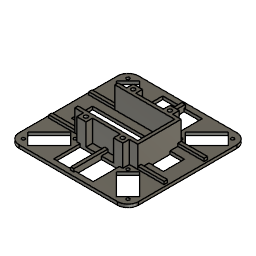
Spider_plate (Autodesk Fusion 360 design; units mm, degrees)
Autodesk Fusion 360 part; units mm, degrees
other "기준 메쉬 피쳐1"
sketch "스케치1" plane through (0, 0, 0) normal (0, 0, 1) x (1, 0, 0)
  line L0 (45.5, -45.5) -> (-45.5, -45.5)
  line L1 (-45.5, -45.5) -> (-45.5, 45.5)
  line L2 (-45.5, 45.5) -> (45.5, 45.5)
  line L3 (45.5, 45.5) -> (45.5, -45.5)
  line L4 (45.5, -45.5) -> (-45.5, 45.5) construction
  line L5 (-45.5, -45.5) -> (45.5, 45.5) construction
  line L6 (15, 41.5) -> (15, 21.5)
  line L7 (-15, 21.5) -> (-15, 41.5)
  line L8 (-1.25, 42.5) -> (1.25, 42.5)
  line L9 (1.25, 42.5) -> (1.25, 16.5)
  line L10 (1.25, 16.5) -> (-1.25, 16.5)
  line L11 (-1.25, 16.5) -> (-1.25, 42.5)
  line L12 (35, -8) -> (-35, -8)
  line L13 (-35, -8) -> (-35, 8)
  line L14 (-35, 8) -> (35, 8)
  line L15 (35, 8) -> (35, -8)
  line L16 (35, -8) -> (-35, 8) construction
  line L17 (-35, -8) -> (35, 8) construction
  line L18 (-15, 41.5) -> (-1.25, 41.5)
  line L19 (1.25, 41.5) -> (15, 41.5)
  line L20 (15, 21.5) -> (1.25, 21.5)
  line L21 (-1.25, 21.5) -> (-15, 21.5)
  line L22 (-44, 16.5) -> (44, 16.5)
  line L23 (44, 16.5) -> (44, 14)
  line L24 (-44, 14) -> (-44, 16.5)
  line L25 (-44, 16.5) -> (44, 16.5)
  line L26 (44, 16.5) -> (44, 14)
  line L27 (-44, 14) -> (-44, 16.5)
  line L28 (-17.4302, 26.1983) -> (-26.1983, 17.4302)
  line L29 (-26.1983, 17.4302) -> (-42.5325, 33.7643)
  line L30 (-42.5325, 33.7643) -> (-33.7643, 42.5325)
  line L31 (-33.7643, 42.5325) -> (-17.4302, 26.1983)
  line L32 (-17.4302, 26.1983) -> (-42.5325, 33.7643) construction
  line L33 (-26.1983, 17.4302) -> (-33.7643, 42.5325) construction
  circle A0 centre (-20.1172, 20.1172) radius 1.2
  circle A1 centre (-39.8455, 39.8455) radius 1.2
  line L34 (42.5325, 33.7643) -> (26.1983, 17.4302)
  line L35 (26.1983, 17.4302) -> (17.4302, 26.1983)
  line L36 (17.4302, 26.1983) -> (33.7643, 42.5325)
  line L37 (33.7643, 42.5325) -> (42.5325, 33.7643)
  circle A2 centre (39.8455, 39.8455) radius 1.2
  circle A3 centre (20.1172, 20.1172) radius 1.2
  line L38 (-24, 16.5) -> (-24, 14)
  line L39 (24, 16.5) -> (24, 14)
  line L40 (-17.5, 16.5) -> (-17.5, 21.5)
  line L41 (-15, 21.5) -> (-17.5, 21.5)
  line L42 (-10.5, 21.5) -> (-10.5, 16.5)
  circle A4 centre (-14, 18) radius 1.5
  line L43 (0, 42.5) -> (0, 16.5)
  line L44 (17.5, 16.5) -> (17.5, 21.5)
  line L45 (10.5, 21.5) -> (10.5, 16.5)
  line L46 (15, 21.5) -> (17.5, 21.5)
  circle A5 centre (14, 18) radius 1.5
  line L47 (-45.5, 0) -> (45.5, 0)
  circle A6 centre (14, -18) radius 1.5
  line L48 (1.25, -42.5) -> (1.25, -16.5)
  line L49 (-17.5, -16.5) -> (-17.5, -21.5)
  line L50 (-17.4302, -26.1983) -> (-42.5325, -33.7643) construction
  line L51 (-10.5, -21.5) -> (-10.5, -16.5)
  line L52 (15, -21.5) -> (17.5, -21.5)
  line L53 (-26.1983, -17.4302) -> (-33.7643, -42.5325) construction
  line L54 (15, -41.5) -> (15, -21.5)
  circle A7 centre (39.8455, -39.8455) radius 1.2
  line L55 (26.1983, -17.4302) -> (17.4302, -26.1983)
  line L56 (42.5325, -33.7643) -> (26.1983, -17.4302)
  line L57 (-17.4302, -26.1983) -> (-26.1983, -17.4302)
  line L58 (-24, -16.5) -> (-24, -14)
  line L59 (17.5, -16.5) -> (17.5, -21.5)
  circle A8 centre (-39.8455, -39.8455) radius 1.2
  line L60 (1.25, -41.5) -> (15, -41.5)
  line L61 (-1.25, -42.5) -> (1.25, -42.5)
  line L62 (-33.7643, -42.5325) -> (-17.4302, -26.1983)
  line L63 (10.5, -21.5) -> (10.5, -16.5)
  circle A9 centre (-14, -18) radius 1.5
  circle A10 centre (-20.1172, -20.1172) radius 1.2
  line L64 (15, -21.5) -> (1.25, -21.5)
  line L65 (-15, -21.5) -> (-15, -41.5)
  line L66 (17.4302, -26.1983) -> (33.7643, -42.5325)
  line L67 (0, -42.5) -> (0, -16.5)
  line L68 (44, -16.5) -> (44, -14)
  circle A11 centre (20.1172, -20.1172) radius 1.2
  line L69 (-1.25, -16.5) -> (-1.25, -42.5)
  line L70 (-44, -14) -> (-44, -16.5)
  line L71 (44, -16.5) -> (44, -14)
  line L72 (33.7643, -42.5325) -> (42.5325, -33.7643)
  line L73 (-26.1983, -17.4302) -> (-42.5325, -33.7643)
  line L74 (24, -16.5) -> (24, -14)
  line L75 (1.25, -16.5) -> (-1.25, -16.5)
  line L76 (-44, -14) -> (-44, -16.5)
  line L77 (-15, -21.5) -> (-17.5, -21.5)
  line L78 (-42.5325, -33.7643) -> (-33.7643, -42.5325)
  line L79 (-44, -16.5) -> (44, -16.5)
  line L80 (-15, -41.5) -> (-1.25, -41.5)
  line L81 (-45.5, -45.5) -> (45.5, -45.5)
  line L82 (-1.25, -21.5) -> (-15, -21.5)
  line L83 (-44, -16.5) -> (44, -16.5)
  line L84 (24, 14) -> (24, -14)
  line L85 (21.5, 14) -> (21.5, -14)
  line L86 (44, 14) -> (24, 14)
  line L87 (21.5, 14) -> (-44, 14)
  line L88 (44, 14) -> (24, 14)
  line L89 (21.5, 14) -> (-44, 14)
  line L90 (44, -14) -> (24, -14)
  line L91 (21.5, -14) -> (-44, -14)
  line L92 (44, -14) -> (24, -14)
  line L93 (21.5, -14) -> (-44, -14)
  point P0 (0, 16.5)
  point P1 (-29.9813, 29.9813)
  point P2 (-29.9813, -29.9813)
  point P3 (0, -16.5)
  dimension "d1" = 91
  dimension "d2" = 91
  dimension "d3" = 30
  dimension "d4" = 20
  dimension "d5" = 2.5
  dimension "d6" = 16
  dimension "d7" = 70
  dimension "d18" = 26
  dimension "d20" = 16.5
  dimension "d21" = 5
  dimension "d27" = 2.5
  dimension "d36" = 1.2
  dimension "d37" = 1.2
  dimension "d42" = 2.4
  dimension "d43" = 2.4
  dimension "d44" = 23.1
  dimension "d45" = 12.4
  dimension "d46" = 42.4
  dimension "d48" = 270
  dimension "d49" = 88
  dimension "d50" = 48
  dimension "d52" = 24
  dimension "d54" = 7
  dimension "d55" = 26.5
  dimension "d56" = 3
  dimension "d57" = 3.5
  dimension "d58" = 2.5
  constraint parallel L1 L3
  constraint coincident L4 origin
  constraint coincident L5 origin
  constraint horizontal L18
  constraint vertical L6
  constraint horizontal L20
  constraint vertical L7
  constraint horizontal L8
  constraint vertical L9
  constraint horizontal L10
  constraint vertical L11
  constraint horizontal L12
  constraint perpendicular L12 L13
  constraint parallel L12 L14
  constraint parallel L13 L15
  constraint coincident L16 origin
  constraint coincident L17 origin
  constraint coincident L11 L18.end
  constraint coincident L9 L19.start
  constraint collinear L18 L19
  constraint coincident L9 L20.end
  constraint coincident L11 L21.start
  constraint collinear L20 L21
  constraint midpoint L10 P0
  constraint vertical origin P0
  constraint equal L20 L21
  constraint horizontal L22
  constraint vertical L23
  constraint horizontal L86
  constraint vertical L24
  constraint horizontal L25
  constraint vertical L26
  constraint horizontal L88
  constraint vertical L27
  constraint vertical L3
  constraint horizontal L2
  constraint horizontal L0
  constraint midpoint P0 L22
  constraint perpendicular L28 L29
  constraint parallel L28 L30
  constraint parallel L29 L31
  constraint coincident L32 P1
  constraint coincident L33 P1
  constraint coincident L4 P1
  constraint coincident L4 A0.centre
  constraint coincident L4 A1.centre
  constraint parallel L4 L29
  constraint coincident L22 L38.start
  constraint coincident L38.end L87
  constraint perpendicular L38 L87
  constraint coincident L25 L39.start
  constraint perpendicular L39 L86
  constraint coincident L22 L40.start
  constraint perpendicular L25 L40
  constraint perpendicular L40 L41
  constraint coincident L21 L42.start
  constraint coincident L25 L42.end
  constraint perpendicular L25 L42
  constraint tangent L25 A4
  constraint midpoint L8 L43.start
  constraint coincident P0 L43.end
  constraint symmetric L7.start L43 L6.end
  constraint symmetric L40.start L43 L44.start
  constraint symmetric L40.end L43 L44.end
  constraint symmetric L42.start L43 L45.start
  constraint symmetric L42.end L43 L45.end
  constraint symmetric A4 L43 A5
  constraint midpoint L1 L47.start
  constraint midpoint L3 L47.end
  constraint symmetric L1.end L47 L0.end
  constraint symmetric L2.end L47 L0.start
  constraint symmetric L7.end L47 L65.end
  constraint symmetric L6.start L47 L54.start
  constraint symmetric L6.end L47 L52.start
  constraint symmetric L7.start L47 L65.start
  constraint symmetric L8.start L47 L61.start
  constraint symmetric L8.end L47 L48.start
  constraint symmetric L9.end L47 L48.end
  constraint symmetric L10.end L47 L69.start
  constraint symmetric L18.end L47 L80.end
  constraint symmetric L19.start L47 L60.start
  constraint symmetric L20.end L47 L64.end
  constraint symmetric L21.start L47 L82.start
  constraint symmetric P0 L47 P3
  constraint symmetric L22.start L47 L70.end
  constraint symmetric L22.end L47 L68.start
  constraint symmetric L23.end L47 L68.end
  constraint symmetric L24.start L47 L70.start
  constraint symmetric L28.start L47 L50.start
  constraint symmetric L28.end L47 L53.start
  constraint symmetric L29.end L47 L50.end
  constraint symmetric L30.end L47 L53.end
  constraint symmetric P1 L47 P2
  constraint symmetric A0 L47 A10
  constraint symmetric A1 L47 A8
  constraint symmetric L34.start L47 L56.start
  constraint symmetric L34.end L47 L55.start
  constraint symmetric L35.end L47 L55.end
  constraint symmetric L36.end L47 L66.end
  constraint symmetric A2 L47 A7
  constraint symmetric A3 L47 A11
  constraint symmetric L38.start L47 L58.start
  constraint symmetric L38.end L47 L58.end
  constraint symmetric L39.start L47 L74.start
  constraint symmetric L39.end L47 L74.end
  constraint symmetric L40.start L47 L49.start
  constraint symmetric L40.end L47 L49.end
  constraint symmetric L42.start L47 L51.start
  constraint symmetric L42.end L47 L51.end
  constraint symmetric A4 L47 A9
  constraint symmetric L43.start L47 L67.start
  constraint symmetric L44.start L47 L59.start
  constraint symmetric L44.end L47 L52.end
  constraint symmetric L45.end L47 L63.end
  constraint symmetric L45.start L47 L63.start
  constraint symmetric A5 L47 A6
  constraint perpendicular L85 L91
  constraint collinear L86 L87
  constraint collinear L88 L89
  constraint collinear L90 L91
  constraint collinear L92 L93
  measures "d1" distance of L0.start L2.end
  measures "d2" distance of L1.end L2.end
  measures "d3" distance of L7.end L6.start
  measures "d4" distance of L7.end L7.start
  measures "d5" distance of L8.start L8.end
  measures "d6" distance of L12.start L14.end
  measures "d7" distance of L12.start L12.end
  measures "d18" distance of L8.end L9.end
  measures "d20" vertical distance of origin L9.end
  measures "d21" distance of L9.end L20.end
  measures "d27" distance of L22.end L23.end
  measures "d36" radius of A0
  measures "d37" radius of A1
  measures "d42" distance of L28 A0.centre
  measures "d43" distance of L30 A1.centre
  measures "d44" distance of L28.start L30.end
  measures "d45" distance of L29.end L30.end
  measures "d46" distance of origin P1
  measures "d49" distance of L23.end L24.start
  measures "d50" distance of L38.start L39.start
  measures "d52" distance of P0 L38.start
  measures "d54" distance of L40 L42
  measures "d55" distance of L22.start L40.start
  measures "d56" diameter of A4
  measures "d57" horizontal distance of L40.start A4.centre
  measures "d58" distance of L84 L85
extrude "돌출1" add sketch "스케치1" along normal blind 2.4 contours L0 L1 L3 L12 L13 L15 L47 L48 L49 L52 L54 L59 L60 L61 L65 L68 L69 L70 L71 L76 L77 L79 L80 L81 L83 L84 L85 L90 L91 L92 L93 | L1 L2 L3 L6 L7 L8 L9 L11 L13 L14 L15 L18 L19 L22 L23 L24 L25 L26 L27 L40 L41 L44 L46 L47 L84 L85 L86 L87 L88 L89 | L9 L20 L22 L25 L45 | L48 L63 L64 L79 L83 | L51 L69 L79 L82 L83 | L11 L21 L22 L25 L42 makes body 1 at (37.5769, -22.5648, 0) makes body 2 at (-7.4167, -18.1667, 0) makes body 3 at (4.3333, -19.8333, 0) makes body 4 at (7.4167, 18.1667, 0) makes body 5 at (-7.4167, 19.8333, 0)
extrude "돌출3" add sketch "스케치1" along normal blind 4.5 separate body contours L22 L23 L25 L26 L39 L86 L88 | L68 L71 L74 L79 L83 L90 L92 | L58 L70 L76 L79 L83 L91 L93 | L22 L24 L25 L27 L38 L87 L89 | L8 L9 L10 L22 L25 L43 | L48 L61 L67 L75 L79 L83 | L8 L10 L11 L22 L25 L43 | L61 L67 L69 L75 L79 L83 makes body 6 at (-37.3333, -16.5, 1.5) makes body 7 at (30.6667, -16.5, 1.5) makes body 8 at (-1.25, -25.1667, 1.5) makes body 9 at (-30.6667, 14, 1.5) makes body 10 at (30.6667, 16.5, 1.5) makes body 11 at (-1.25, 25.1667, 1.5)
extrude "돌출4" add sketch "스케치1" along normal blind 19 separate body contours L12 L47 L84 L85 | L14 L47 L84 L85 | L10 L14 L22 L25 L38 L39 L84 L85 L87 L89 | L12 L58 L74 L75 L79 L83 L84 L85 L91 L93 makes body 12
fillet "필렛1" radius 8 4 edges at (45.5, -45.5, 1.2) (45.5, 45.5, 1.2) (-45.5, 45.5, 1.2) (-45.5, -45.5, 1.2) on bodies 1
extrude "돌출5" add sketch "스케치1" along normal blind 19 contours L20 L22 L25 L44 L45 L46 | L52 L59 L63 L64 L79 L83 | L49 L51 L77 L79 L82 L83 | L21 L22 L25 L40 L41 L42 bodies 1 10 8 11 7 6 9 12 2 3 4 5
extrude "돌출2" [suppressed]
